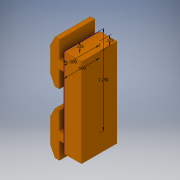
# Autodesk Inventor part: 2020liftconecter
Saved by Autodesk Inventor 2017 (Build 210142000, 142)
## iProperties
Created: 2017-12-06
Part Number: 2020liftconecter
Material: Generic
Document SubType Name: Modeling
Designer: User
Density: 1 g/cm^3
Appearance: Default(1)
Author: User
Autodesk Inventor part; units mm, degrees
ref_plane "YZ Plane" through (0, 0, 0) normal (1, 0, 0) x (0, 1, 0)
ref_plane "XZ Plane" through (0, 0, 0) normal (0, 1, 0) x (-1, 0, 0)
sketch "Sketch1" plane through (0, 0, 0) normal (1, 0, 0) x (0, 1, 0)
  line L0 (0, 0) -> (31.75, 0)
  line L1 (31.75, 0) -> (31.75, -12.7)
  line L2 (31.75, -12.7) -> (0, -12.7)
  line L3 (0, -12.7) -> (0, 0)
  line L4 (28.575, 0) -> (25.4, 0)
  line L5 (25.4, 0) -> (25.4, -12.7)
  line L6 (25.4, -12.7) -> (28.575, -12.7)
  line L7 (28.575, -12.7) -> (28.575, 0)
  dimension "d0" = 31.75
  dimension "d1" = 12.7
  dimension "d4" = 3.175
  dimension "d5" = 12.7
  dimension "d6" = 3.175
  constraints: 16 end point, 4 parallel, 2 horizontal, 2 perpendicular, 1 point on line
  measures "d0" distance of L1.end L2.end
  measures "d1" distance between parallel lines of L0 L2
  measures "d4" distance of L6.end L5.end
  measures "d5" distance between parallel lines of L0 L6
  measures "d6" distance between parallel lines of L1 L7
extrude "Extrusion1" add sketch "Sketch1" along normal blind 6.35
extrude "Extrusion2" add sketch "Sketch1" against normal blind 1.5875 contours L0 L7 L2 L5
sketch "Sketch2" plane through (-1.5875, 0, 0) normal (-1, 0, 0) x (0, 0, 1)
  line L0 (-12.7, 34.671) -> (0, 34.671)
  line L1 (0, 34.671) -> (0, 19.304)
  line L2 (0, 19.304) -> (-12.7, 19.304)
  line L3 (-12.7, 19.304) -> (-12.7, 34.671)
  line L4 (-12.7, 31.75) -> (-12.7, 28.575) projected
  line L5 (-12.7, 25.4) -> (0, 25.4) projected
  line L6 (0, 28.575) -> (-12.7, 28.575) projected
  point P0 (0, 0)
  dimension "d9" = 12.7
  dimension "d10" = 0
  dimension "d11" = 6.096
  dimension "d12" = 6.096
  constraints: 8 end point, 2 parallel, 1 horizontal, 1 perpendicular
  measures "d9" distance of L0.start L0.end
  measures "d10" distance between parallel lines of L3 L4
  measures "d11" distance between parallel lines of L2 L5
  measures "d12" distance between parallel lines of L6 L0
extrude "Extrusion3" add sketch "Sketch2" along normal blind 3.175
sketch "Sketch3" plane through (0, 0, 0) normal (0, 0, 1) x (1, 0, 0)
  line L0 (-4.7625, 34.671) -> (-4.7625, 31.496)
  line L1 (-4.7625, 19.304) -> (-4.7625, 34.671) projected
  line L2 (-1.5875, 34.671) -> (-1.5875, 28.575) projected
  line L3 (-1.5875, 34.671) -> (-3.1623, 34.671)
  line L4 (-1.5875, 34.671) -> (-4.7625, 34.671) projected
  line L5 (-1.5875, 19.304) -> (-3.1623, 19.304)
  line L6 (-1.5875, 19.304) -> (-4.7625, 19.304) projected
  line L7 (-4.7625, 19.304) -> (-4.7625, 22.479)
  line L8 (-4.7625, 22.479) -> (-3.1623, 19.304)
  line L9 (-4.7625, 19.304) -> (-3.1623, 19.304)
  line L10 (-4.7625, 31.496) -> (-3.1623, 34.671)
  line L11 (-4.7625, 34.671) -> (-3.1623, 34.671)
  point P0 (0, 0)
  dimension "d16" = 3.175
  dimension "d17" = 1.5748
  dimension "d18" = 1.5748
  dimension "d19" = 3.175
  constraints: 16 end point, 4 point on line, 1 collinear, 1 horizontal
  measures "d16" distance of L0.start L0.end
  measures "d17" distance of L2.start L3.end
  measures "d18" distance of L5.start L5.end
  measures "d19" distance of L1.start L7.end
extrude "Extrusion4" cut sketch "Sketch3" against normal through all
ref_plane "Work Plane3" through (0, 15.875, 0) normal (0, 1, 0) x (1, 0, 0)
mirror "Mirror1" about plane through (0, 15.875, 0) normal (0, 1, 0) of "Extrusion2", "Extrusion3", "Extrusion4"
equation "\"d5\" = d1"
equation "\"d9\" = d1"
body "Solid1"
